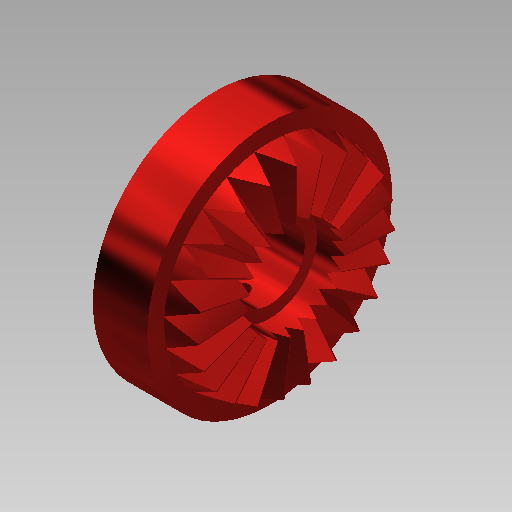
# Autodesk Inventor part: pad
Saved by Autodesk Inventor 2018.1 (Build 221171000, 171)
## iProperties
Created: 2013-08-26
Part Number: pad
Material: Generic
Document SubType Name: Modeling
Designer: Konstantin
Density: 1 g/cm^3
Appearance: Default
Mass: 1.11009 g
Surface Area: 10.0445 cm^2
Volume: 1.11009 cm^3
Author: Konstantin
Autodesk Inventor part; units mm, degrees
ref_plane "XZ Plane" through (0, 0, 0) normal (0, 1, 0) x (-1, 0, 0)
ref_plane "XY Plane" through (0, 0, 0) normal (0, 0, 1) x (1, 0, 0)
sketch "Sketch1" plane through (0, 0, 0) normal (0, 0, 1) x (1, 0, 0)
  line L0 (0, 0) -> (6, 0)
  line L1 (6, 0) -> (6, 7.25)
  line L2 (4, 9) -> (0, 9)
  line L3 (0, 9) -> (0, 0)
  line L4 (4, 9) -> (4, 7.75)
  line L5 (4, 7.75) -> (6, 7.25)
  constraints: 12 end point, 2 horizontal, 2 parallel, 2 vertical, 1 perpendicular, 1 other
revolve "Revolution1" add sketch "Sketch1" angle 360 about axis through (0, 0, 0) along (1, 0, 0)
sketch "Sketch3" plane through (6, 0, 0) normal (1, 0, 0) x (0, 0, -1)
  line L0 (0, 0) -> (0, 9)
  line L1 (0, 0) -> (2.3294, 8.6933)
  arc A0 (2.3294, 8.6933) -> (0, 9) centre (0, 0) ccw
  constraints: 4 end point, 2 point on circle, 2 vertical, 1 centre point, 2 other
extrude "Extrusion2" cut sketch "Sketch3" against normal blind 2 draft -26
pattern_circular "Circular Pattern1" count 23 over 360 about axis through (-10, 0, 0) along (1, 0, 0) of "Extrusion2"
sketch "Sketch4" plane through (0, 0, 0) normal (-1, 0, 0) x (0, 0, 1)
  circle A0 centre (0, 0) radius 2.6
  dimension "d17" = 5.2
  constraints: 1 centre point, 1 coincident
  measures "d17" diameter of A0
extrude "Extrusion3" cut sketch "Sketch4" against normal blind 10
ref_plane "Work Plane2" through (6, 0, 0) normal (1, 0, 0) x (0, 1, 0)
sketch "Sketch5" plane through (6, 0, 0) normal (1, 0, 0) x (0, 1, 0)
  circle A0 centre (0, 0) radius 3.5
  dimension "d21" = 7
  constraints: 1 centre point, 1 coincident
  measures "d21" diameter of A0
extrude "Extrusion4" cut sketch "Sketch5" against normal blind 2
sketch "Sketch6" plane through (0, 0, 0) normal (0, 1, 0) x (-1, 0, 0)
  circle A0 centre (-2, 0) radius 0.5
  constraints: 1 centre point, 1 other
extrude "Extrusion5" cut sketch "Sketch6" against normal blind 4
body "Solid1"
